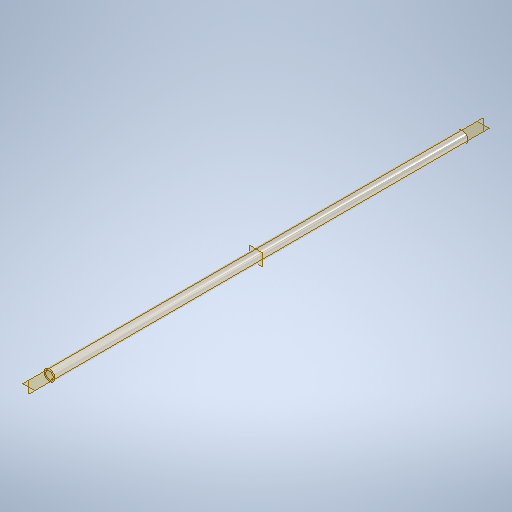
# Autodesk Inventor part: Peça8_perna
Saved by Autodesk Inventor 2025.2 (Build 292293000, 293)
## iProperties
Created: 2025-03-28
Part Number: Peça8_perna
Material: Aço
Document SubType Name: Modeling
Designer: Formação
Density: 7.85 g/cm^3
Appearance: Titânio - Polido
Author: Formação
Autodesk Inventor part; units mm, degrees
sketch "Esboço2" plane through (0, 0, 0) normal (0, 0, 1) x (1, 0, 0)
  circle A0 centre (0, 0) radius 10
  circle A1 centre (0, 0) radius 7
  dimension "d2" = 20
  dimension "d3" = 3
  constraints: 2 centre point, 2 coincident, 1 concentric
  measures "d2" diameter of A0
  measures "d3" radial gap between concentric circles of A0 A1
extrude "Extrusão1" add sketch "Esboço2" along normal mid plane 750
